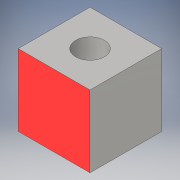
# Autodesk Inventor part: P4_1PivotCube
Saved by Autodesk Inventor 2016 (Build 200138000, 138)
## iProperties
Created: 2016-02-09
Part Number: P4_1PivotCube
Material: Generic
Document SubType Name: Modeling
Designer: choueugene
Density: 1 g/cm^3
Appearance: Default
Author: choueugene
Autodesk Inventor part; units mm, degrees
ref_plane "YZ Plane" through (0, 0, 0) normal (1, 0, 0) x (0, 1, 0)
ref_plane "XZ Plane" through (0, 0, 0) normal (0, 1, 0) x (-1, 0, 0)
ref_plane "XY Plane" through (0, 0, 0) normal (0, 0, 1) x (1, 0, 0)
sketch "SquareSketch1" plane through (0, 0, 0) normal (0, 1, 0) x (-1, 0, 0)
  line L0 (0, 0) -> (6.35, 0)
  line L1 (6.35, 0) -> (6.35, -6.35)
  line L2 (6.35, -6.35) -> (0, -6.35)
  line L3 (0, -6.35) -> (0, 0)
  point P0 (3.175, -3.175)
  point P1 (6.35, -3.175)
  point P2 (3.175, -6.35)
  dimension "d0" = 6.35
  dimension "d1" = 6.35
  constraints: 8 end point, 2 midpoint, 2 parallel, 1 horizontal, 1 horizontal alignment, 1 perpendicular, 1 vertical alignment
  measures "d0" distance of L0.end L1.end
  measures "d1" distance of L0.start L0.end
extrude "CubeExtrusion1" add sketch "SquareSketch1" along normal blind 6.35
hole "Hole1" at (-3.175, 0, -3.175) direction (0, 1, 0) diameter 2.54 end through all
equation "\"d1\" = d0"
equation "\"d2\" = d0"
body "Solid1"
